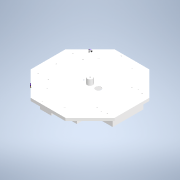
# Autodesk Inventor part: trail 2
Saved by Autodesk Inventor 2020.2 (Build 242310000, 310)
## iProperties
Created: 2020-02-13
Part Number: trail 2
Material: PAEK Plastic
Document SubType Name: Modeling
Designer: lenovo
Density: 1.32 g/cm^3
Appearance: Smooth - White
Author: lenovo
Autodesk Inventor part; units mm, degrees
ref_plane "YZ Plane" through (0, 0, 0) normal (1, 0, 0) x (0, 1, 0)
ref_plane "XZ Plane" through (0, 0, 0) normal (0, 1, 0) x (-1, 0, 0)
ref_plane "XY Plane" through (0, 0, 0) normal (0, 0, 1) x (1, 0, 0)
sketch "Sketch1" plane through (0, 0, 0) normal (0, 1, 0) x (-1, 0, 0)
  line L0 (62.7534, 151.5) -> (151.5, 62.7534)
  line L1 (151.5, 62.7534) -> (151.5, -62.7534)
  line L2 (151.5, -62.7534) -> (62.7534, -151.5)
  line L3 (62.7534, -151.5) -> (-62.7534, -151.5)
  line L4 (-62.7534, -151.5) -> (-151.5, -62.7534)
  line L5 (-151.5, -62.7534) -> (-151.5, 62.7534)
  line L6 (-151.5, 62.7534) -> (-62.7534, 151.5)
  line L7 (-62.7534, 151.5) -> (62.7534, 151.5)
  point P0 (0, 0)
  point P1 (0, 0)
  dimension "d0" = 303
  constraints: 16 end point, 1 coincident, 17 other
  measures "d0" distance between parallel lines of L3 L7
extrude "Extrusion1" add sketch "Sketch1" along normal blind 10
sketch "Sketch2" plane through (0, 10, 0) normal (0, 1, 0) x (1, 0, 0)
  circle A0 centre (-125, -62.5) radius 2
  circle A1 centre (-88, -62.5) radius 2
  line L0 (-151.5, 62.7534) -> (-151.5, -62.7534) projected
  line L1 (151.5, -62.7534) -> (151.5, 62.7534) projected
  line L2 (-62.7534, -151.5) -> (62.7534, -151.5) projected
  line L3 (62.7534, 151.5) -> (-62.7534, 151.5) projected
  circle A2 centre (-125, 62.5) radius 2
  circle A3 centre (-88, 62.5) radius 2
  circle A4 centre (125, -62.5) radius 2
  circle A5 centre (88, -62.5) radius 2
  circle A6 centre (125, 62.5) radius 2
  circle A7 centre (88, 62.5) radius 2
  point P0 (0, 0)
  dimension "d3" = 4
  dimension "d4" = 4
  constraints: 8 centre point
  measures "d3" diameter of A0
  measures "d4" diameter of A1
extrude "Extrusion2" cut sketch "Sketch2" along normal mid plane 30
sketch "Sketch3" plane through (0, 10, 0) normal (0, 1, 0) x (1, 0, 0)
  circle A0 centre (0, 0) radius 10
  circle A1 centre (0, 0) radius 2.5
  dimension "d7" = 20
  dimension "d8" = 5
  constraints: 2 centre point, 2 coincident
  measures "d7" diameter of A0
  measures "d8" diameter of A1
extrude "Extrusion3" add sketch "Sketch3" along normal blind 20
sketch "Sketch4" plane through (0, 0, 0) normal (0, -1, 0) x (1, 0, 0)
  line L0 (-151.5, -62.7534) -> (-151.5, 62.7534) projected
  line L1 (151.5, 62.7534) -> (151.5, -62.7534) projected
  line L2 (77, -55) -> (137, -55)
  line L3 (137, -55) -> (137, 55)
  line L4 (137, 55) -> (77, 55)
  line L5 (77, 55) -> (77, -55)
  line L6 (77, -55) -> (137, 55) construction
  line L7 (137, -55) -> (77, 55) construction
  line L8 (-2.5, 110) -> (62.5, 110)
  line L9 (62.5, 110) -> (62.5, -110)
  line L10 (62.5, -110) -> (-2.5, -110)
  line L11 (-2.5, -110) -> (-2.5, 110)
  line L12 (-2.5, 110) -> (62.5, -110) construction
  line L13 (62.5, 110) -> (-2.5, -110) construction
  line L14 (-110, 50) -> (-10, 50)
  line L15 (-10, 50) -> (-10, -50)
  line L16 (-10, -50) -> (-110, -50)
  line L17 (-110, -50) -> (-110, 50)
  line L18 (-110, 50) -> (-10, -50) construction
  line L19 (-10, 50) -> (-110, -50) construction
  line L20 (-10, -55) -> (-50, -55)
  line L21 (-50, -55) -> (-50, -130)
  line L22 (-50, -130) -> (-10, -130)
  line L23 (-10, -130) -> (-10, -55)
  line L24 (-10, 55) -> (-50, 55)
  line L25 (-50, 55) -> (-50, 130)
  line L26 (-50, 130) -> (-10, 130)
  line L27 (-10, 130) -> (-10, 55)
  point P0 (0, 0)
  point P1 (107, 0)
  point P2 (30, 0)
  point P3 (-60, 0)
  dimension "d11" = 303
  dimension "d12" = 60
  dimension "d13" = 110
  dimension "d14" = 65
  dimension "d15" = 220
  dimension "d16" = 100
  dimension "d17" = 100
  dimension "d18" = 40
  dimension "d19" = 75
  dimension "d20" = 75
  constraints: 52 end point, 10 parallel, 6 midpoint, 5 horizontal, 5 perpendicular, 2 point on line
  measures "d11" distance between parallel lines of L0 L1
  measures "d12" distance of L4.end L3.end
  measures "d13" distance of L3.end L2.end
  measures "d14" distance of L9.end L10.end
  measures "d15" distance of L8.end L9.end
  measures "d16" distance of L15.end L16.end
  measures "d17" distance of L14.end L15.end
  measures "d18" distance of L22.end L21.end
  measures "d19" distance of L21.end L20.end
  measures "d20" distance of L24.end L25.end
extrude "Extrusion4" add sketch "Sketch4" along normal blind 50
shell "Shell1" thickness 1 removed faces 5 at (-36.6667, -50, -80) at (117, -50, -18.3333) at (19.1667, -50, 36.6667) at (-76.6667, -50, 16.6667) at (-36.6667, -50, 105)
sketch "Sketch5" plane through (0, -50, 0) normal (0, -1, 0) x (1, 0, 0)
  line L0 (136, -54) -> (78, -54)
  line L1 (78, -54) -> (78, 54)
  line L2 (78, 54) -> (136, 54)
  line L3 (136, 54) -> (136, -54)
  line L4 (136, -54) -> (78, 54) construction
  line L5 (78, -54) -> (136, 54) construction
  line L6 (-11, 49) -> (-109, 49)
  line L7 (-109, 49) -> (-109, -49)
  line L8 (-109, -49) -> (-11, -49)
  line L9 (-11, -49) -> (-11, 49)
  line L10 (-11, 49) -> (-109, -49) construction
  line L11 (-109, 49) -> (-11, -49) construction
  line L12 (-49, -56) -> (-11, -56)
  line L13 (-11, -56) -> (-11, -129)
  line L14 (-11, -129) -> (-49, -129)
  line L15 (-49, -129) -> (-49, -56)
  line L16 (-49, -56) -> (-11, -129) construction
  line L17 (-11, -56) -> (-49, -129) construction
  line L18 (-49, 56) -> (-11, 56) projected
  line L19 (-49, 129) -> (-11, 129)
  line L20 (-11, 129) -> (-11, 56)
  line L21 (-11, 56) -> (-49, 56)
  line L22 (-49, 56) -> (-49, 129)
  line L23 (-49, 129) -> (-11, 56) construction
  line L24 (-11, 129) -> (-49, 56) construction
  point P0 (0, 0)
  point P1 (107, 0)
  point P2 (-60, 0)
  point P3 (-30, -92.5)
  point P4 (-30, 92.5)
  dimension "d24" = 58
  dimension "d25" = 108
  dimension "d26" = 98
  dimension "d27" = 98
  dimension "d28" = 38
  dimension "d29" = 73
  dimension "d30" = 38
  dimension "d31" = 73
  constraints: 48 end point, 8 midpoint, 8 parallel, 4 horizontal, 4 perpendicular
  measures "d24" distance of L1.end L2.end
  measures "d25" distance of L0.end L1.end
  measures "d26" distance of L8.end L7.end
  measures "d27" distance of L7.end L6.end
  measures "d28" distance of L13.end L14.end
  measures "d29" distance of L12.end L13.end
  measures "d30" distance of L18.end L21.end
  measures "d31" distance of L19.end L18.end
extrude "Extrusion5" cut sketch "Sketch5" against normal blind 50
sketch "Sketch6" plane through (61.5, -50, -109) normal (-1, 0, 0) x (0, 0, 1)
  point P0 (109, 50)
  point P1 (69.2464, 26.2759)
hole "Hole1" at (61.5, -23.7241, -39.7536) direction (1, 0, 0) diameter 20 depth 30
sketch "Sketch7" plane through (61.5, -50, -109) normal (-1, 0, 0) x (0, 0, 1)
  circle A0 centre (69.2464, 26.2759) radius 10 projected
  circle A1 centre (69.2464, 26.2759) radius 10
  circle A2 centre (69.2464, 26.2759) radius 11
  point P0 (109, 50)
  dimension "d41" = 20
  dimension "d42" = 22
  constraints: 2 centre point, 2 coincident
  measures "d41" diameter of A1
  measures "d42" diameter of A2
extrude "Extrusion6" add sketch "Sketch7" against normal blind 16.25
sketch "Sketch8" plane through (-11, -50, -56) normal (-1, 0, 0) x (0, 0, 1)
  point P0 (56, 50)
  point P1 (-23.9194, 17.1128)
  point P2 (139.049, 18.9509)
hole "Hole2" at (-11, -32.8872, -79.9194) at (-11, -31.0491, 83.049) direction (1, 0, 0) diameter 10 depth 30
sketch "Sketch9" plane through (-50, 0, -130) normal (-1, 0, 0) x (0, 0, 1)
  point P0 (130, 0)
  point P1 (36.6302, -24.6866)
  point P2 (221.0681, -25.2267)
hole "Hole3" at (-50, -24.6866, -93.3698) at (-50, -25.2267, 91.0681) direction (1, 0, 0) diameter 10 depth 3
sketch "Sketch10" plane through (-49, 1, 56) normal (0, 0, 1) x (1, 0, 0)
  point P0 (49, -1)
  point P1 (20.3131, -27.2211)
hole "Hole4" at (-28.6869, -26.2211, 56) direction (0, 0, -1) diameter 12.5 depth 30
sketch "Sketch11" plane through (-109, 1, -49) normal (0, 0, 1) x (1, 0, 0)
  point P0 (109, -1)
  point P1 (78.9333, -26.6179)
hole "Hole5" at (-30.0667, -25.6179, -49) direction (0, 0, -1) diameter 12.5 depth 30
sketch "Sketch12" plane through (-49, 1, 56) normal (0, 0, 1) x (1, 0, 0)
  circle A0 centre (20.3131, -27.2211) radius 6.25 projected
  circle A1 centre (20.3131, -27.2211) radius 6.25
  circle A2 centre (20.3131, -27.2211) radius 6.25 projected
  circle A3 centre (20.3131, -27.2211) radius 6.75
  point P0 (49, -1)
  dimension "d73" = 13.5
  constraints: 2 centre point, 2 coincident
  measures "d73" diameter of A3
extrude "Extrusion7" add sketch "Sketch12" against normal blind 7
sketch "Sketch13" plane through (-11, 1, -56) normal (0, 0, -1) x (-1, 0, 0)
  circle A0 centre (19.0667, -26.6179) radius 6.25 projected
  circle A1 centre (19.0667, -26.6179) radius 6.75
  point P0 (-11, -1)
  dimension "d76" = 13.5
  constraints: 1 centre point, 1 coincident
  measures "d76" diameter of A1
extrude "Extrusion8" add sketch "Sketch13" against normal blind 7
sketch "Sketch14" plane through (-62.3391, 9, 150.5) normal (0, -1, 0) x (1, 0, 0)
  circle A0 centre (92.34, -150.5) radius 10
  point P0 (62.3391, -150.5)
  dimension "d79" = 20
  constraints: 1 centre point
  measures "d79" diameter of A0
extrude "Extrusion9" cut sketch "Sketch14" against normal blind 10
sketch "Sketch15" plane through (-11, -50, 129) normal (-1, 0, 0) x (0, 0, 1)
  circle A0 centre (-45.951, 18.9509) radius 5 projected
  circle A1 centre (-45.951, 18.9509) radius 5
  circle A2 centre (-45.951, 18.9509) radius 5.5
  circle A3 centre (-208.9194, 17.1128) radius 5 projected
  circle A4 centre (-208.9194, 17.1128) radius 5
  circle A5 centre (-208.9194, 17.1128) radius 5.5
  point P0 (-129, 50)
  dimension "d82" = 11
  dimension "d83" = 11
  constraints: 4 centre point, 4 coincident
  measures "d82" diameter of A2
  measures "d83" diameter of A5
extrude "Extrusion10" add sketch "Sketch15" against normal blind 9.5
sketch "Sketch16" plane through (0, -50, 0) normal (0, -1, 0) x (1, 0, 0)
  line L0 (160.7646, -155.9788) -> (-160.7646, -155.9788)
  line L1 (-160.7646, -155.9788) -> (-160.7646, 155.9788)
  line L2 (-160.7646, 155.9788) -> (160.7646, 155.9788)
  line L3 (160.7646, 155.9788) -> (160.7646, -155.9788)
  circle A0 centre (0, 0) radius 10 projected
  line L4 (160.7646, -155.9788) -> (-160.7646, 155.9788) construction
  line L5 (-160.7646, -155.9788) -> (160.7646, 155.9788) construction
  constraints: 12 end point, 2 midpoint, 2 parallel, 1 horizontal, 1 perpendicular
extrude "Extrusion11" cut sketch "Sketch16" against normal blind 20
sketch "Sketch17" plane through (-151.5, 0, -62.7534) normal (-0.7071, 0, -0.7071) x (-0.7071, 0, 0.7071)
  circle A0 centre (-62.7534, 5) radius 5
  point P0 (-62.7534, 0)
  dimension "d88" = 10
  constraints: 1 centre point
  measures "d88" diameter of A0
sketch "Sketch18" plane through (-62.7534, 0, 151.5) normal (-0.7071, 0, 0.7071) x (0.7071, 0, 0.7071)
  circle A0 centre (-62.7534, 5) radius 5
  point P0 (-62.7534, 0)
  dimension "d89" = 10
  constraints: 1 centre point
  measures "d89" diameter of A0
sketch "Sketch19" plane through (0, 0, 0) normal (0, -1, 0) x (1, 0, 0)
  circle A0 centre (0, 0) radius 2.5
  circle A1 centre (-22.9979, 0) radius 2
  circle A2 centre (107, -67) radius 2
  circle A3 centre (-122, 0) radius 2
  circle A4 centre (-62, -92.5) radius 2
  circle A5 centre (-30, -142) radius 2
  circle A6 centre (30, -122) radius 2
  line L0 (157.9023, 0) -> (-166.1221, 0)
  circle A7 centre (-22.9979, 0) radius 2
  circle A8 centre (107, 67) radius 2
  circle A9 centre (-122, 0) radius 2
  circle A10 centre (-62, 92.5) radius 2
  circle A11 centre (-30, 142) radius 2
  circle A12 centre (30, 122) radius 2
  dimension "d90" = 4
  dimension "d91" = 4
  dimension "d92" = 4
  dimension "d93" = 4
  dimension "d94" = 4
  dimension "d95" = 4
  constraints: 13 centre point, 4 symmetric about line, 2 end point, 1 coincident, 1 horizontal, 6 other
  measures "d90" diameter of A1
  measures "d91" diameter of A2
  measures "d92" diameter of A3
  measures "d93" diameter of A4
  measures "d94" diameter of A5
  measures "d95" diameter of A6
extrude "Extrusion12" cut sketch "Sketch19" against normal blind 10
sketch "Sketch20" plane through (0, 10, 0) normal (0, 1, 0) x (1, 0, 0)
  circle A0 centre (0, 0) radius 10 projected
  circle A1 centre (0, 0) radius 10
  circle A2 centre (0, 0) radius 2.5
  constraints: 2 centre point, 2 coincident
extrude "Extrusion13" add sketch "Sketch20" along normal blind 20
sketch "Sketch21" plane through (0, 9, 0) normal (0, -1, 0) x (1, 0, 0)
  circle A0 centre (0, 0) radius 2.5
  circle A1 centre (0, 0) radius 2.5 projected
  circle A2 centre (0, 0) radius 9
  constraints: 2 centre point, 2 coincident
extrude "Extrusion14" add sketch "Sketch21" against normal blind 2
sketch "Sketch22" plane through (0, 10, 0) normal (0, 1, 0) x (1, 0, 0)
  circle A0 centre (0, 140) radius 2
  circle A1 centre (0, -140) radius 2
  circle A2 centre (50, -140) radius 2
  circle A3 centre (50, 140) radius 2
  point P0 (0, 0)
  dimension "d102" = 4
  dimension "d103" = 4
  dimension "d104" = 4
  dimension "d105" = 4
  constraints: 4 centre point
  measures "d102" diameter of A0
  measures "d103" diameter of A1
  measures "d104" diameter of A2
  measures "d105" diameter of A3
extrude "Extrusion15" cut sketch "Sketch22" against normal blind 10
body "Solid1"
